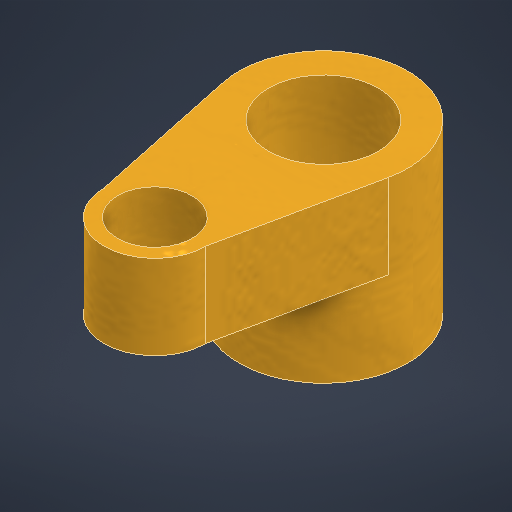
# Autodesk Inventor part: Palanca_potenciometro
Saved by Autodesk Inventor 2027 (Build 310192060, 192F)
## iProperties
Created: 2026-06-11
Part Number: Palanca_potenciometro
Material: Genérico
Document SubType Name: Modeling
Designer: angel
Density: 1 g/cm^3
Appearance: Soldadura - Latón
Author: angel
Autodesk Inventor part; units mm, degrees
ref_plane "YZ Plane" through (0, 0, 0) normal (1, 0, 0) x (0, 1, 0)
ref_plane "XZ Plane" through (0, 0, 0) normal (0, 1, 0) x (-1, 0, 0)
ref_plane "XY Plane" through (0, 0, 0) normal (0, 0, 1) x (1, 0, 0)
sketch "Boceto1" plane through (0, 0, 0) normal (0, 1, 0) x (-1, 0, 0)
  circle A0 centre (0, 0) radius 3.25
  circle A1 centre (0, 0) radius 5
  line L0 (0, 13) -> (0, 10)
  circle A2 centre (0, 10) radius 3
  circle A3 centre (0, 10) radius 2.2
  line L1 (3, 10) -> (4.8923, 1.0323)
  line L2 (-3, 10) -> (-4.8923, 1.0323)
  dimension "d0" = 6.5
  dimension "d1" = 10
  dimension "d3" = 3
  dimension "d4" = 4.4
  dimension "d7" = 10
  dimension "d15" = 8.9677
  dimension "d16" = 8.9677
  dimension "d17" = 3
  constraints: 6 end point, 5 point on circle, 4 centre point, 4 coincident, 2 tangent
  measures "d0" diameter of A0
  measures "d1" diameter of A1
  measures "d3" distance of L0.start L0.end
  measures "d4" diameter of A3
  measures "d7" distance of point (0, 0) L0.end
  measures "d15" vertical distance of L2.start L2.end
  measures "d16" vertical distance of L1.start L1.end
  measures "d17" distance of L0.start L0.end
extrude "Extrusión3" add sketch "Boceto1" along normal blind 5
extrude "Extrusión4" add sketch "Boceto1" against normal blind 5 contours A1
